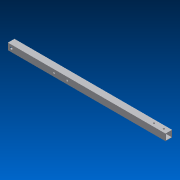
# Autodesk Inventor part: ArmBAr
Saved by Autodesk Inventor 2013 (Build 170138000, 138)
## iProperties
Created: 2013-07-15
Part Number: ArmBAr
Material: Aluminum 6061
Document SubType Name: Modeling
Designer: root
Density: 1 g/cm^3
Author: root
Autodesk Inventor part; units mm, degrees
ref_plane "YZ Plane" through (0, 0, 0) normal (1, 0, 0) x (0, 1, 0)
ref_plane "XZ Plane" through (0, 0, 0) normal (0, 1, 0) x (-1, 0, 0)
ref_plane "XY Plane" through (0, 0, 0) normal (0, 0, 1) x (1, 0, 0)
sketch "Sketch1" plane through (0, 0, 0) normal (1, 0, 0) x (0, 1, 0)
  line L0 (0, 0) -> (25.4, 0)
  line L1 (25.4, 0) -> (25.4, 25.4)
  line L2 (25.4, 25.4) -> (0, 25.4)
  line L3 (0, 25.4) -> (0, 0)
  line L4 (1.651, 23.749) -> (23.749, 23.749)
  line L5 (23.749, 23.749) -> (23.749, 1.651)
  line L6 (23.749, 1.651) -> (1.651, 1.651)
  line L7 (1.651, 1.651) -> (1.651, 23.749)
  dimension "d0" = 25.4
  dimension "d2" = 25.4
  dimension "d3" = 1.651
  dimension "d5" = 1.651
  dimension "d6" = 1.651
  dimension "d7" = 1.651
  constraints: 16 end point, 4 parallel, 2 horizontal, 2 perpendicular
  measures "d0" distance of L1.end L2.end
  measures "d2" distance of L2.end L0.start
  measures "d3" distance between parallel lines of L5 L1
  measures "d5" distance between parallel lines of L2 L4
  measures "d6" distance between parallel lines of L3 L7
  measures "d7" distance between parallel lines of L0 L6
extrude "Extrusion1" add sketch "Sketch1" along normal blind 609.6
sketch "Sketch2" plane through (0, 0, 25.4) normal (0, 0, 1) x (1, 0, 0)
  line L0 (0, 25.4) -> (0, 0) projected
  line L1 (0, 25.4) -> (609.6, 25.4) projected
  point P0 (12.7, 12.7)
  dimension "d10" = 12.7
  dimension "d11" = 12.7
  measures "d10" distance from line of point (12.7, 12.7) L1
  measures "d11" distance from line of point (12.7, 12.7) L0
hole "Hole1" at (12.7, 12.7, 25.4) direction (0, 0, -1) diameter 9.525 end through all
sketch "Sketch3" plane through (0, 25.4, 25.4) normal (0, 1, 0) x (1, 0, 0)
  line L0 (609.6, 25.4) -> (609.6, 0) projected
  point P0 (590.55, 12.7)
  point P1 (552.45, 12.7)
  dimension "d19" = 19.05
  dimension "d20" = 38.1
  measures "d19" distance from line of point (590.55, 12.7) L0
  measures "d20" distance of point (590.55, 12.7) point (552.45, 12.7)
hole "Hole2" at (590.55, 25.4, 12.7) at (552.45, 25.4, 12.7) direction (0, -1, 0) diameter 6.35 end through all
sketch "Sketch4" plane through (0, 0, 25.4) normal (0, 0, 1) x (1, 0, 0)
  line L0 (0, 25.4) -> (0, 0) projected
  line L1 (0, 0) -> (609.6, 0) projected
  line L2 (0, 25.4) -> (609.6, 25.4) projected
  point P0 (177.8, 12.7)
  point P1 (228.6, 12.7)
  dimension "d28" = 177.8
  dimension "d29" = 12.7
  dimension "d37" = 12.7
  dimension "d38" = 50.8
  measures "d28" distance from line of L0 point (177.8, 12.7)
  measures "d29" distance from line of L1 point (177.8, 12.7)
  measures "d37" distance from line of L2 point (228.6, 12.7)
  measures "d38" distance of point (177.8, 12.7) point (228.6, 12.7)
hole "Hole3" at (177.8, 12.7, 25.4) at (228.6, 12.7, 25.4) direction (0, 0, -1) diameter 6.35 end through all
body "Solid1"
